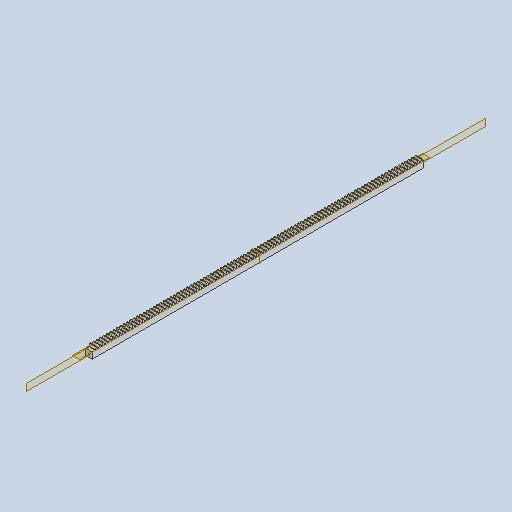
# Autodesk Inventor part: Zahnradbahn
Saved by Autodesk Inventor 2024 (Build 280153000, 153)
## iProperties
Created: 2022-05-05
Part Number: Zahnradbahn
Material: Generisch
Document SubType Name: Modeling
Designer: 123St
Density: 1 g/cm^3
Appearance: Vorgabe
Mass: 12.6552 g
Surface Area: 103.602 cm^2
Volume: 12.6552 cm^3
Zahnbreite: 1,700 mm
Teilung: 3,142 mm
Fussrundung: 0,380 mm
Modul: 1,000 mm
Kopfspiel: 0,100 mm
Zaehnezahl_1: 98,000 oE
Author: 123St
Autodesk Inventor part; units mm, degrees
(part 1 of 2)
ref_plane "YZ Plane" through (0, 0, 0) normal (1, 0, 0) x (0, 1, 0)
ref_plane "XZ Plane" through (0, 0, 0) normal (0, 1, 0) x (-1, 0, 0)
sketch "Skizze1" plane through (0, 0, 0) normal (1, 0, 0) x (0, 1, 0)
  line L0 (3.4, 153.938) -> (-3.4, 153.938)
  line L1 (-3.4, 153.938) -> (-3.4, -153.938)
  line L2 (-3.4, -153.938) -> (3.4, -153.938)
  line L3 (3.4, -153.938) -> (3.4, 153.938)
  line L4 (3.4, 153.938) -> (-3.4, -153.938) construction
  line L5 (-3.4, 153.938) -> (3.4, -153.938) construction
  point P0 (0, 0)
  dimension "d0" = 6.8
  dimension "d1" = 307.8761
  constraints: 12 end point, 2 midpoint, 2 parallel, 1 horizontal, 1 perpendicular
  measures "d0" distance of L0.start L0.end
  measures "d1" distance of L2.end L0.start
extrude "Extrusion1" add sketch "Skizze1" along normal blind 6
sketch "Skizze3" plane through (0, -3.4, -153.938) normal (0, -1, 0) x (1, 0, 0)
  line L0 (0, 307.8761) -> (6, 307.8761)
  line L1 (6, 307.8761) -> (6, 0)
  line L2 (6, 0) -> (0, 0)
  line L3 (0, 0) -> (0, 307.8761)
  line L4 (6, 307.8761) -> (6, 0) construction
  line L5 (0, 307.8761) -> (6, 307.8761) projected
  line L6 (0, 0) -> (0, 307.8761) construction
  line L7 (6, 0) -> (6, 307.8761) construction
  point P0 (0, 153.938)
  dimension "d21" = 307.8761
  dimension "d24" = 0
  constraints: 8 end point, 2 collinear, 2 parallel, 1 horizontal, 1 perpendicular
  measures "d21" distance of L0.end L1.end
  measures "d24" distance between parallel lines of L5 L0
extrude "Extrusion3" add sketch "Skizze3" along normal blind 2.5
sketch "Skizze5" plane through (6, 0, 0) normal (1, 0, 0) x (0, 0, -1)
  line L0 (-153.938, 3.4) -> (-153.938, -5.9) construction
  line L1 (-153.938, 0) -> (153.938, 0) construction
  line L2 (153.938, -5.9) -> (-153.938, -5.9) construction
  line L3 (-153.938, 0) -> (-153.686, 0)
  arc A0 (-153.686, 0) -> (-153.5075, 0.125) centre (-153.686, 0.19) ccw
  line L4 (-153.5075, 0.125) -> (-152.7887, 2.1)
  line L5 (-152.7887, 2.1) -> (-151.9458, 2.1)
  line L6 (-151.9458, 2.1) -> (-151.227, 0.125)
  arc A1 (-151.227, 0.125) -> (-151.0484, 0) centre (-151.0484, 0.19) ccw
  line L7 (-151.0484, 0) -> (-150.7964, 0)
  line L8 (-152.3672, 2.1) -> (-152.3672, 0) construction
  line L9 (-153.686, 0) -> (-151.0484, 0) construction
  line L10 (-153.1526, 1.1) -> (-151.5818, 1.1) construction
  line L11 (-147.9068, 0) -> (-147.6549, 0)
  arc A2 (-148.0854, 0.125) -> (-147.9068, 0) centre (-147.9068, 0.19) ccw
  line L12 (-150.011, 1.1) -> (-148.4403, 1.1) construction
  line L13 (-150.3659, 0.125) -> (-149.6471, 2.1)
  line L14 (-148.8042, 2.1) -> (-148.0854, 0.125)
  line L15 (-149.2257, 2.1) -> (-149.2257, 0) construction
  line L16 (-149.6471, 2.1) -> (-148.8042, 2.1)
  line L17 (-150.5445, 0) -> (-147.9068, 0) construction
  arc A3 (-150.5445, 0) -> (-150.3659, 0.125) centre (-150.5445, 0.19) ccw
  line L18 (-150.7964, 0) -> (-150.5445, 0)
  line L19 (-144.7653, 0) -> (-144.5133, 0)
  arc A4 (-144.9438, 0.125) -> (-144.7653, 0) centre (-144.7653, 0.19) ccw
  line L20 (-146.8695, 1.1) -> (-145.2987, 1.1) construction
  line L21 (-147.2243, 0.125) -> (-146.5055, 2.1)
  line L22 (-145.6626, 2.1) -> (-144.9438, 0.125)
  line L23 (-146.0841, 2.1) -> (-146.0841, 0) construction
  line L24 (-146.5055, 2.1) -> (-145.6626, 2.1)
  line L25 (-147.4029, 0) -> (-144.7653, 0) construction
  arc A5 (-147.4029, 0) -> (-147.2243, 0.125) centre (-147.4029, 0.19) ccw
  line L26 (-147.6549, 0) -> (-147.4029, 0)
  line L27 (-141.6237, 0) -> (-141.3717, 0)
  arc A6 (-141.8022, 0.125) -> (-141.6237, 0) centre (-141.6237, 0.19) ccw
  line L28 (-143.7279, 1.1) -> (-142.1571, 1.1) construction
  line L29 (-144.0827, 0.125) -> (-143.3639, 2.1)
  line L30 (-142.521, 2.1) -> (-141.8022, 0.125)
  line L31 (-142.9425, 2.1) -> (-142.9425, 0) construction
  line L32 (-143.3639, 2.1) -> (-142.521, 2.1)
  line L33 (-144.2613, 0) -> (-141.6237, 0) construction
  arc A7 (-144.2613, 0) -> (-144.0827, 0.125) centre (-144.2613, 0.19) ccw
  line L34 (-144.5133, 0) -> (-144.2613, 0)
  line L35 (-138.4821, 0) -> (-138.2301, 0)
  arc A8 (-138.6606, 0.125) -> (-138.4821, 0) centre (-138.4821, 0.19) ccw
  line L36 (-140.5863, 1.1) -> (-139.0155, 1.1) construction
  line L37 (-140.9411, 0.125) -> (-140.2223, 2.1)
  line L38 (-139.3794, 2.1) -> (-138.6606, 0.125)
  line L39 (-139.8009, 2.1) -> (-139.8009, 0) construction
  line L40 (-140.2223, 2.1) -> (-139.3794, 2.1)
  line L41 (-141.1197, 0) -> (-138.4821, 0) construction
  arc A9 (-141.1197, 0) -> (-140.9411, 0.125) centre (-141.1197, 0.19) ccw
  line L42 (-141.3717, 0) -> (-141.1197, 0)
  line L43 (-135.3405, 0) -> (-135.0885, 0)
  arc A10 (-135.519, 0.125) -> (-135.3405, 0) centre (-135.3405, 0.19) ccw
  line L44 (-137.4447, 1.1) -> (-135.8739, 1.1) construction
  line L45 (-137.7995, 0.125) -> (-137.0807, 2.1)
  line L46 (-136.2379, 2.1) -> (-135.519, 0.125)
  line L47 (-136.6593, 2.1) -> (-136.6593, 0) construction
  line L48 (-137.0807, 2.1) -> (-136.2379, 2.1)
  line L49 (-137.9781, 0) -> (-135.3405, 0) construction
  arc A11 (-137.9781, 0) -> (-137.7995, 0.125) centre (-137.9781, 0.19) ccw
  line L50 (-138.2301, 0) -> (-137.9781, 0)
  line L51 (-132.1989, 0) -> (-131.9469, 0)
  arc A12 (-132.3774, 0.125) -> (-132.1989, 0) centre (-132.1989, 0.19) ccw
  line L52 (-134.3031, 1.1) -> (-132.7323, 1.1) construction
  line L53 (-134.658, 0.125) -> (-133.9391, 2.1)
  line L54 (-133.0963, 2.1) -> (-132.3774, 0.125)
  line L55 (-133.5177, 2.1) -> (-133.5177, 0) construction
  line L56 (-133.9391, 2.1) -> (-133.0963, 2.1)
  line L57 (-134.8365, 0) -> (-132.1989, 0) construction
  arc A13 (-134.8365, 0) -> (-134.658, 0.125) centre (-134.8365, 0.19) ccw
  line L58 (-135.0885, 0) -> (-134.8365, 0)
  line L59 (-129.0573, 0) -> (-128.8053, 0)
  arc A14 (-129.2358, 0.125) -> (-129.0573, 0) centre (-129.0573, 0.19) ccw
  line L60 (-131.1615, 1.1) -> (-129.5907, 1.1) construction
  line L61 (-131.5164, 0.125) -> (-130.7975, 2.1)
  line L62 (-129.9547, 2.1) -> (-129.2358, 0.125)
  line L63 (-130.3761, 2.1) -> (-130.3761, 0) construction
  line L64 (-130.7975, 2.1) -> (-129.9547, 2.1)
  line L65 (-131.6949, 0) -> (-129.0573, 0) construction
  arc A15 (-131.6949, 0) -> (-131.5164, 0.125) centre (-131.6949, 0.19) ccw
  line L66 (-131.9469, 0) -> (-131.6949, 0)
  line L67 (-125.9157, 0) -> (-125.6637, 0)
  arc A16 (-126.0942, 0.125) -> (-125.9157, 0) centre (-125.9157, 0.19) ccw
  line L68 (-128.0199, 1.1) -> (-126.4491, 1.1) construction
  line L69 (-128.3748, 0.125) -> (-127.6559, 2.1)
  line L70 (-126.8131, 2.1) -> (-126.0942, 0.125)
  line L71 (-127.2345, 2.1) -> (-127.2345, 0) construction
  line L72 (-127.6559, 2.1) -> (-126.8131, 2.1)
  line L73 (-128.5533, 0) -> (-125.9157, 0) construction
  arc A17 (-128.5533, 0) -> (-128.3748, 0.125) centre (-128.5533, 0.19) ccw
  line L74 (-128.8053, 0) -> (-128.5533, 0)
  line L75 (-122.7741, 0) -> (-122.5221, 0)
  arc A18 (-122.9526, 0.125) -> (-122.7741, 0) centre (-122.7741, 0.19) ccw
  line L76 (-124.8783, 1.1) -> (-123.3075, 1.1) construction
  line L77 (-125.2332, 0.125) -> (-124.5143, 2.1)
  line L78 (-123.6715, 2.1) -> (-122.9526, 0.125)
  line L79 (-124.0929, 2.1) -> (-124.0929, 0) construction
  line L80 (-124.5143, 2.1) -> (-123.6715, 2.1)
  line L81 (-125.4117, 0) -> (-122.7741, 0) construction
  arc A19 (-125.4117, 0) -> (-125.2332, 0.125) centre (-125.4117, 0.19) ccw
  line L82 (-125.6637, 0) -> (-125.4117, 0)
  line L83 (-119.6325, 0) -> (-119.3805, 0)
  arc A20 (-119.8111, 0.125) -> (-119.6325, 0) centre (-119.6325, 0.19) ccw
  line L84 (-121.7367, 1.1) -> (-120.1659, 1.1) construction
  line L85 (-122.0916, 0.125) -> (-121.3727, 2.1)
  line L86 (-120.5299, 2.1) -> (-119.8111, 0.125)
  line L87 (-120.9513, 2.1) -> (-120.9513, 0) construction
  line L88 (-121.3727, 2.1) -> (-120.5299, 2.1)
  line L89 (-122.2701, 0) -> (-119.6325, 0) construction
  arc A21 (-122.2701, 0) -> (-122.0916, 0.125) centre (-122.2701, 0.19) ccw
  line L90 (-122.5221, 0) -> (-122.2701, 0)
  line L91 (-116.4909, 0) -> (-116.2389, 0)
  arc A22 (-116.6695, 0.125) -> (-116.4909, 0) centre (-116.4909, 0.19) ccw
  line L92 (-118.5951, 1.1) -> (-117.0243, 1.1) construction
  line L93 (-118.95, 0.125) -> (-118.2312, 2.1)
  line L94 (-117.3883, 2.1) -> (-116.6695, 0.125)
  line L95 (-117.8097, 2.1) -> (-117.8097, 0) construction
  line L96 (-118.2312, 2.1) -> (-117.3883, 2.1)
  line L97 (-119.1285, 0) -> (-116.4909, 0) construction
  arc A23 (-119.1285, 0) -> (-118.95, 0.125) centre (-119.1285, 0.19) ccw
  line L98 (-119.3805, 0) -> (-119.1285, 0)
  line L99 (-113.3493, 0) -> (-113.0973, 0)
  arc A24 (-113.5279, 0.125) -> (-113.3493, 0) centre (-113.3493, 0.19) ccw
  line L100 (-115.4535, 1.1) -> (-113.8827, 1.1) construction
  line L101 (-115.8084, 0.125) -> (-115.0896, 2.1)
  line L102 (-114.2467, 2.1) -> (-113.5279, 0.125)
  line L103 (-114.6681, 2.1) -> (-114.6681, 0) construction
  line L104 (-115.0896, 2.1) -> (-114.2467, 2.1)
  line L105 (-115.9869, 0) -> (-113.3493, 0) construction
  arc A25 (-115.9869, 0) -> (-115.8084, 0.125) centre (-115.9869, 0.19) ccw
  line L106 (-116.2389, 0) -> (-115.9869, 0)
  line L107 (-110.2077, 0) -> (-109.9557, 0)
  arc A26 (-110.3863, 0.125) -> (-110.2077, 0) centre (-110.2077, 0.19) ccw
  line L108 (-112.3119, 1.1) -> (-110.7411, 1.1) construction
  line L109 (-112.6668, 0.125) -> (-111.948, 2.1)
  line L110 (-111.1051, 2.1) -> (-110.3863, 0.125)
  line L111 (-111.5265, 2.1) -> (-111.5265, 0) construction
  line L112 (-111.948, 2.1) -> (-111.1051, 2.1)
  line L113 (-112.8453, 0) -> (-110.2077, 0) construction
  arc A27 (-112.8453, 0) -> (-112.6668, 0.125) centre (-112.8453, 0.19) ccw
  line L114 (-113.0973, 0) -> (-112.8453, 0)
  line L115 (-107.0661, 0) -> (-106.8142, 0)
  arc A28 (-107.2447, 0.125) -> (-107.0661, 0) centre (-107.0661, 0.19) ccw
  line L116 (-109.1703, 1.1) -> (-107.5995, 1.1) construction
  line L117 (-109.5252, 0.125) -> (-108.8064, 2.1)
  line L118 (-107.9635, 2.1) -> (-107.2447, 0.125)
  line L119 (-108.3849, 2.1) -> (-108.3849, 0) construction
  line L120 (-108.8064, 2.1) -> (-107.9635, 2.1)
  line L121 (-109.7038, 0) -> (-107.0661, 0) construction
  arc A29 (-109.7038, 0) -> (-109.5252, 0.125) centre (-109.7038, 0.19) ccw
  line L122 (-109.9557, 0) -> (-109.7038, 0)
  line L123 (-103.9245, 0) -> (-103.6726, 0)
  arc A30 (-104.1031, 0.125) -> (-103.9245, 0) centre (-103.9245, 0.19) ccw
  line L124 (-106.0288, 1.1) -> (-104.458, 1.1) construction
  line L125 (-106.3836, 0.125) -> (-105.6648, 2.1)
  line L126 (-104.8219, 2.1) -> (-104.1031, 0.125)
  line L127 (-105.2434, 2.1) -> (-105.2434, 0) construction
  line L128 (-105.6648, 2.1) -> (-104.8219, 2.1)
  line L129 (-106.5622, 0) -> (-103.9245, 0) construction
  arc A31 (-106.5622, 0) -> (-106.3836, 0.125) centre (-106.5622, 0.19) ccw
  line L130 (-106.8142, 0) -> (-106.5622, 0)
  line L131 (-100.783, 0) -> (-100.531, 0)
  arc A32 (-100.9615, 0.125) -> (-100.783, 0) centre (-100.783, 0.19) ccw
  line L132 (-102.8872, 1.1) -> (-101.3164, 1.1) construction
  line L133 (-103.242, 0.125) -> (-102.5232, 2.1)
  line L134 (-101.6803, 2.1) -> (-100.9615, 0.125)
  line L135 (-102.1018, 2.1) -> (-102.1018, 0) construction
  line L136 (-102.5232, 2.1) -> (-101.6803, 2.1)
  line L137 (-103.4206, 0) -> (-100.783, 0) construction
  arc A33 (-103.4206, 0) -> (-103.242, 0.125) centre (-103.4206, 0.19) ccw
  line L138 (-103.6726, 0) -> (-103.4206, 0)
  line L139 (-97.6414, 0) -> (-97.3894, 0)
  arc A34 (-97.8199, 0.125) -> (-97.6414, 0) centre (-97.6414, 0.19) ccw
  line L140 (-99.7456, 1.1) -> (-98.1748, 1.1) construction
  line L141 (-100.1004, 0.125) -> (-99.3816, 2.1)
  line L142 (-98.5387, 2.1) -> (-97.8199, 0.125)
  line L143 (-98.9602, 2.1) -> (-98.9602, 0) construction
  line L144 (-99.3816, 2.1) -> (-98.5387, 2.1)
  line L145 (-100.279, 0) -> (-97.6414, 0) construction
  arc A35 (-100.279, 0) -> (-100.1004, 0.125) centre (-100.279, 0.19) ccw
  line L146 (-100.531, 0) -> (-100.279, 0)
  line L147 (-94.4998, 0) -> (-94.2478, 0)
  arc A36 (-94.6783, 0.125) -> (-94.4998, 0) centre (-94.4998, 0.19) ccw
  line L148 (-96.604, 1.1) -> (-95.0332, 1.1) construction
  line L149 (-96.9588, 0.125) -> (-96.24, 2.1)
  line L150 (-95.3971, 2.1) -> (-94.6783, 0.125)
  line L151 (-95.8186, 2.1) -> (-95.8186, 0) construction
  line L152 (-96.24, 2.1) -> (-95.3971, 2.1)
  line L153 (-97.1374, 0) -> (-94.4998, 0) construction
  arc A37 (-97.1374, 0) -> (-96.9588, 0.125) centre (-97.1374, 0.19) ccw
  line L154 (-97.3894, 0) -> (-97.1374, 0)
  line L155 (-91.3582, 0) -> (-91.1062, 0)
  arc A38 (-91.5367, 0.125) -> (-91.3582, 0) centre (-91.3582, 0.19) ccw
  line L156 (-93.4624, 1.1) -> (-91.8916, 1.1) construction
  line L157 (-93.8172, 0.125) -> (-93.0984, 2.1)
  line L158 (-92.2556, 2.1) -> (-91.5367, 0.125)
  line L159 (-92.677, 2.1) -> (-92.677, 0) construction
  line L160 (-93.0984, 2.1) -> (-92.2556, 2.1)
  line L161 (-93.9958, 0) -> (-91.3582, 0) construction
  arc A39 (-93.9958, 0) -> (-93.8172, 0.125) centre (-93.9958, 0.19) ccw
  line L162 (-94.2478, 0) -> (-93.9958, 0)
  line L163 (-88.2166, 0) -> (-87.9646, 0)
  arc A40 (-88.3951, 0.125) -> (-88.2166, 0) centre (-88.2166, 0.19) ccw
  line L164 (-90.3208, 1.1) -> (-88.75, 1.1) construction
  line L165 (-90.6757, 0.125) -> (-89.9568, 2.1)
  line L166 (-89.114, 2.1) -> (-88.3951, 0.125)
  line L167 (-89.5354, 2.1) -> (-89.5354, 0) construction
  line L168 (-89.9568, 2.1) -> (-89.114, 2.1)
  line L169 (-90.8542, 0) -> (-88.2166, 0) construction
  arc A41 (-90.8542, 0) -> (-90.6757, 0.125) centre (-90.8542, 0.19) ccw
  line L170 (-91.1062, 0) -> (-90.8542, 0)
  line L171 (-85.075, 0) -> (-84.823, 0)
  arc A42 (-85.2535, 0.125) -> (-85.075, 0) centre (-85.075, 0.19) ccw
  line L172 (-87.1792, 1.1) -> (-85.6084, 1.1) construction
  line L173 (-87.5341, 0.125) -> (-86.8152, 2.1)
  line L174 (-85.9724, 2.1) -> (-85.2535, 0.125)
  line L175 (-86.3938, 2.1) -> (-86.3938, 0) construction
  line L176 (-86.8152, 2.1) -> (-85.9724, 2.1)
  line L177 (-87.7126, 0) -> (-85.075, 0) construction
  arc A43 (-87.7126, 0) -> (-87.5341, 0.125) centre (-87.7126, 0.19) ccw
  line L178 (-87.9646, 0) -> (-87.7126, 0)
  line L179 (-81.9334, 0) -> (-81.6814, 0)
  arc A44 (-82.1119, 0.125) -> (-81.9334, 0) centre (-81.9334, 0.19) ccw
  line L180 (-84.0376, 1.1) -> (-82.4668, 1.1) construction
  line L181 (-84.3925, 0.125) -> (-83.6736, 2.1)
  line L182 (-82.8308, 2.1) -> (-82.1119, 0.125)
  line L183 (-83.2522, 2.1) -> (-83.2522, 0) construction
  line L184 (-83.6736, 2.1) -> (-82.8308, 2.1)
  line L185 (-84.571, 0) -> (-81.9334, 0) construction
  arc A45 (-84.571, 0) -> (-84.3925, 0.125) centre (-84.571, 0.19) ccw
  line L186 (-84.823, 0) -> (-84.571, 0)
  line L187 (-78.7918, 0) -> (-78.5398, 0)
  arc A46 (-78.9703, 0.125) -> (-78.7918, 0) centre (-78.7918, 0.19) ccw
  line L188 (-80.896, 1.1) -> (-79.3252, 1.1) construction
  line L189 (-81.2509, 0.125) -> (-80.532, 2.1)
  line L190 (-79.6892, 2.1) -> (-78.9703, 0.125)
  line L191 (-80.1106, 2.1) -> (-80.1106, 0) construction
  line L192 (-80.532, 2.1) -> (-79.6892, 2.1)
  line L193 (-81.4294, 0) -> (-78.7918, 0) construction
  arc A47 (-81.4294, 0) -> (-81.2509, 0.125) centre (-81.4294, 0.19) ccw
  line L194 (-81.6814, 0) -> (-81.4294, 0)
  line L195 (-75.6502, 0) -> (-75.3982, 0)
  arc A48 (-75.8288, 0.125) -> (-75.6502, 0) centre (-75.6502, 0.19) ccw
  line L196 (-77.7544, 1.1) -> (-76.1836, 1.1) construction
  line L197 (-78.1093, 0.125) -> (-77.3904, 2.1)
  line L198 (-76.5476, 2.1) -> (-75.8288, 0.125)
  line L199 (-76.969, 2.1) -> (-76.969, 0) construction
  line L200 (-77.3904, 2.1) -> (-76.5476, 2.1)
  line L201 (-78.2878, 0) -> (-75.6502, 0) construction
  arc A49 (-78.2878, 0) -> (-78.1093, 0.125) centre (-78.2878, 0.19) ccw
  line L202 (-78.5398, 0) -> (-78.2878, 0)
  line L203 (-72.5086, 0) -> (-72.2566, 0)
  arc A50 (-72.6872, 0.125) -> (-72.5086, 0) centre (-72.5086, 0.19) ccw
  line L204 (-74.6128, 1.1) -> (-73.042, 1.1) construction
  line L205 (-74.9677, 0.125) -> (-74.2489, 2.1)
  line L206 (-73.406, 2.1) -> (-72.6872, 0.125)
  line L207 (-73.8274, 2.1) -> (-73.8274, 0) construction
  line L208 (-74.2489, 2.1) -> (-73.406, 2.1)
  line L209 (-75.1462, 0) -> (-72.5086, 0) construction
  arc A51 (-75.1462, 0) -> (-74.9677, 0.125) centre (-75.1462, 0.19) ccw
  line L210 (-75.3982, 0) -> (-75.1462, 0)
  line L211 (-69.367, 0) -> (-69.115, 0)
  arc A52 (-69.5456, 0.125) -> (-69.367, 0) centre (-69.367, 0.19) ccw
  line L212 (-71.4712, 1.1) -> (-69.9004, 1.1) construction
  line L213 (-71.8261, 0.125) -> (-71.1073, 2.1)
  line L214 (-70.2644, 2.1) -> (-69.5456, 0.125)
  line L215 (-70.6858, 2.1) -> (-70.6858, 0) construction
  line L216 (-71.1073, 2.1) -> (-70.2644, 2.1)
  line L217 (-72.0046, 0) -> (-69.367, 0) construction
  arc A53 (-72.0046, 0) -> (-71.8261, 0.125) centre (-72.0046, 0.19) ccw
  line L218 (-72.2566, 0) -> (-72.0046, 0)
  line L219 (-66.2254, 0) -> (-65.9734, 0)
  arc A54 (-66.404, 0.125) -> (-66.2254, 0) centre (-66.2254, 0.19) ccw
  line L220 (-68.3296, 1.1) -> (-66.7588, 1.1) construction
  line L221 (-68.6845, 0.125) -> (-67.9657, 2.1)
  line L222 (-67.1228, 2.1) -> (-66.404, 0.125)
  line L223 (-67.5442, 2.1) -> (-67.5442, 0) construction
  line L224 (-67.9657, 2.1) -> (-67.1228, 2.1)
  line L225 (-68.863, 0) -> (-66.2254, 0) construction
  arc A55 (-68.863, 0) -> (-68.6845, 0.125) centre (-68.863, 0.19) ccw
  line L226 (-69.115, 0) -> (-68.863, 0)
  line L227 (-63.0838, 0) -> (-62.8319, 0)
  arc A56 (-63.2624, 0.125) -> (-63.0838, 0) centre (-63.0838, 0.19) ccw
  line L228 (-65.188, 1.1) -> (-63.6173, 1.1) construction
  line L229 (-65.5429, 0.125) -> (-64.8241, 2.1)
  line L230 (-63.9812, 2.1) -> (-63.2624, 0.125)
  line L231 (-64.4026, 2.1) -> (-64.4026, 0) construction
  line L232 (-64.8241, 2.1) -> (-63.9812, 2.1)
  line L233 (-65.7215, 0) -> (-63.0838, 0) construction
  arc A57 (-65.7215, 0) -> (-65.5429, 0.125) centre (-65.7215, 0.19) ccw
  line L234 (-65.9734, 0) -> (-65.7215, 0)
  line L235 (-59.9423, 0) -> (-59.6903, 0)
  arc A58 (-60.1208, 0.125) -> (-59.9423, 0) centre (-59.9423, 0.19) ccw
  line L236 (-62.0465, 1.1) -> (-60.4757, 1.1) construction
  line L237 (-62.4013, 0.125) -> (-61.6825, 2.1)
  line L238 (-60.8396, 2.1) -> (-60.1208, 0.125)
  line L239 (-61.2611, 2.1) -> (-61.2611, 0) construction
  line L240 (-61.6825, 2.1) -> (-60.8396, 2.1)
  line L241 (-62.5799, 0) -> (-59.9423, 0) construction
  arc A59 (-62.5799, 0) -> (-62.4013, 0.125) centre (-62.5799, 0.19) ccw
  line L242 (-62.8319, 0) -> (-62.5799, 0)
  line L243 (-56.8007, 0) -> (-56.5487, 0)
  arc A60 (-56.9792, 0.125) -> (-56.8007, 0) centre (-56.8007, 0.19) ccw
  line L244 (-58.9049, 1.1) -> (-57.3341, 1.1) construction
  line L245 (-59.2597, 0.125) -> (-58.5409, 2.1)
  line L246 (-57.698, 2.1) -> (-56.9792, 0.125)
  line L247 (-58.1195, 2.1) -> (-58.1195, 0) construction
  line L248 (-58.5409, 2.1) -> (-57.698, 2.1)
  line L249 (-59.4383, 0) -> (-56.8007, 0) construction
  arc A61 (-59.4383, 0) -> (-59.2597, 0.125) centre (-59.4383, 0.19) ccw
  line L250 (-59.6903, 0) -> (-59.4383, 0)
  line L251 (-53.6591, 0) -> (-53.4071, 0)
  arc A62 (-53.8376, 0.125) -> (-53.6591, 0) centre (-53.6591, 0.19) ccw
  line L252 (-55.7633, 1.1) -> (-54.1925, 1.1) construction
  line L253 (-56.1181, 0.125) -> (-55.3993, 2.1)
  line L254 (-54.5564, 2.1) -> (-53.8376, 0.125)
  line L255 (-54.9779, 2.1) -> (-54.9779, 0) construction
  line L256 (-55.3993, 2.1) -> (-54.5564, 2.1)
  line L257 (-56.2967, 0) -> (-53.6591, 0) construction
  arc A63 (-56.2967, 0) -> (-56.1181, 0.125) centre (-56.2967, 0.19) ccw
  line L258 (-56.5487, 0) -> (-56.2967, 0)
  line L259 (-50.5175, 0) -> (-50.2655, 0)
  arc A64 (-50.696, 0.125) -> (-50.5175, 0) centre (-50.5175, 0.19) ccw
  line L260 (-52.6217, 1.1) -> (-51.0509, 1.1) construction
  line L261 (-52.9765, 0.125) -> (-52.2577, 2.1)
  line L262 (-51.4149, 2.1) -> (-50.696, 0.125)
  line L263 (-51.8363, 2.1) -> (-51.8363, 0) construction
  line L264 (-52.2577, 2.1) -> (-51.4149, 2.1)
  line L265 (-53.1551, 0) -> (-50.5175, 0) construction
  arc A65 (-53.1551, 0) -> (-52.9765, 0.125) centre (-53.1551, 0.19) ccw
  line L266 (-53.4071, 0) -> (-53.1551, 0)
  line L267 (-47.3759, 0) -> (-47.1239, 0)
  arc A66 (-47.5544, 0.125) -> (-47.3759, 0) centre (-47.3759, 0.19) ccw
  line L268 (-49.4801, 1.1) -> (-47.9093, 1.1) construction
  line L269 (-49.8349, 0.125) -> (-49.1161, 2.1)
  line L270 (-48.2733, 2.1) -> (-47.5544, 0.125)
  line L271 (-48.6947, 2.1) -> (-48.6947, 0) construction
  line L272 (-49.1161, 2.1) -> (-48.2733, 2.1)
  line L273 (-50.0135, 0) -> (-47.3759, 0) construction
  arc A67 (-50.0135, 0) -> (-49.8349, 0.125) centre (-50.0135, 0.19) ccw
  line L274 (-50.2655, 0) -> (-50.0135, 0)
  line L275 (-44.2343, 0) -> (-43.9823, 0)
  arc A68 (-44.4128, 0.125) -> (-44.2343, 0) centre (-44.2343, 0.19) ccw
  line L276 (-46.3385, 1.1) -> (-44.7677, 1.1) construction
  line L277 (-46.6934, 0.125) -> (-45.9745, 2.1)
  line L278 (-45.1317, 2.1) -> (-44.4128, 0.125)
  line L279 (-45.5531, 2.1) -> (-45.5531, 0) construction
  line L280 (-45.9745, 2.1) -> (-45.1317, 2.1)
  line L281 (-46.8719, 0) -> (-44.2343, 0) construction
  arc A69 (-46.8719, 0) -> (-46.6934, 0.125) centre (-46.8719, 0.19) ccw
  line L282 (-47.1239, 0) -> (-46.8719, 0)
  line L283 (-41.0927, 0) -> (-40.8407, 0)
  arc A70 (-41.2712, 0.125) -> (-41.0927, 0) centre (-41.0927, 0.19) ccw
  line L284 (-43.1969, 1.1) -> (-41.6261, 1.1) construction
  line L285 (-43.5518, 0.125) -> (-42.8329, 2.1)
  line L286 (-41.9901, 2.1) -> (-41.2712, 0.125)
  line L287 (-42.4115, 2.1) -> (-42.4115, 0) construction
  line L288 (-42.8329, 2.1) -> (-41.9901, 2.1)
  line L289 (-43.7303, 0) -> (-41.0927, 0) construction
  arc A71 (-43.7303, 0) -> (-43.5518, 0.125) centre (-43.7303, 0.19) ccw
  line L290 (-43.9823, 0) -> (-43.7303, 0)
  line L291 (-37.9511, 0) -> (-37.6991, 0)
  arc A72 (-38.1296, 0.125) -> (-37.9511, 0) centre (-37.9511, 0.19) ccw
  line L292 (-40.0553, 1.1) -> (-38.4845, 1.1) construction
  line L293 (-40.4102, 0.125) -> (-39.6913, 2.1)
  line L294 (-38.8485, 2.1) -> (-38.1296, 0.125)
  line L295 (-39.2699, 2.1) -> (-39.2699, 0) construction
  line L296 (-39.6913, 2.1) -> (-38.8485, 2.1)
  line L297 (-40.5887, 0) -> (-37.9511, 0) construction
  arc A73 (-40.5887, 0) -> (-40.4102, 0.125) centre (-40.5887, 0.19) ccw
  line L298 (-40.8407, 0) -> (-40.5887, 0)
  line L299 (-34.8095, 0) -> (-34.5575, 0)
  arc A74 (-34.9881, 0.125) -> (-34.8095, 0) centre (-34.8095, 0.19) ccw
  line L300 (-36.9137, 1.1) -> (-35.3429, 1.1) construction
  line L301 (-37.2686, 0.125) -> (-36.5497, 2.1)
  line L302 (-35.7069, 2.1) -> (-34.9881, 0.125)
  line L303 (-36.1283, 2.1) -> (-36.1283, 0) construction
  line L304 (-36.5497, 2.1) -> (-35.7069, 2.1)
  line L305 (-37.4471, 0) -> (-34.8095, 0) construction
  arc A75 (-37.4471, 0) -> (-37.2686, 0.125) centre (-37.4471, 0.19) ccw
  line L306 (-37.6991, 0) -> (-37.4471, 0)
  line L307 (-31.6679, 0) -> (-31.4159, 0)
  arc A76 (-31.8465, 0.125) -> (-31.6679, 0) centre (-31.6679, 0.19) ccw
  line L308 (-33.7721, 1.1) -> (-32.2013, 1.1) construction
  line L309 (-34.127, 0.125) -> (-33.4082, 2.1)
  line L310 (-32.5653, 2.1) -> (-31.8465, 0.125)
  line L311 (-32.9867, 2.1) -> (-32.9867, 0) construction
  line L312 (-33.4082, 2.1) -> (-32.5653, 2.1)
  line L313 (-34.3055, 0) -> (-31.6679, 0) construction
  arc A77 (-34.3055, 0) -> (-34.127, 0.125) centre (-34.3055, 0.19) ccw
  line L314 (-34.5575, 0) -> (-34.3055, 0)
  line L315 (-28.5263, 0) -> (-28.2743, 0)
  arc A78 (-28.7049, 0.125) -> (-28.5263, 0) centre (-28.5263, 0.19) ccw
  line L316 (-30.6305, 1.1) -> (-29.0597, 1.1) construction
  line L317 (-30.9854, 0.125) -> (-30.2666, 2.1)
  line L318 (-29.4237, 2.1) -> (-28.7049, 0.125)
  line L319 (-29.8451, 2.1) -> (-29.8451, 0) construction
  line L320 (-30.2666, 2.1) -> (-29.4237, 2.1)
  line L321 (-31.1639, 0) -> (-28.5263, 0) construction
  arc A79 (-31.1639, 0) -> (-30.9854, 0.125) centre (-31.1639, 0.19) ccw
  line L322 (-31.4159, 0) -> (-31.1639, 0)
  line L323 (-25.3847, 0) -> (-25.1327, 0)
  arc A80 (-25.5633, 0.125) -> (-25.3847, 0) centre (-25.3847, 0.19) ccw
  line L324 (-27.4889, 1.1) -> (-25.9181, 1.1) construction
  line L325 (-27.8438, 0.125) -> (-27.125, 2.1)
  line L326 (-26.2821, 2.1) -> (-25.5633, 0.125)
  line L327 (-26.7035, 2.1) -> (-26.7035, 0) construction
  line L328 (-27.125, 2.1) -> (-26.2821, 2.1)
  line L329 (-28.0223, 0) -> (-25.3847, 0) construction
  arc A81 (-28.0223, 0) -> (-27.8438, 0.125) centre (-28.0223, 0.19) ccw
  line L330 (-28.2743, 0) -> (-28.0223, 0)
  line L331 (-22.2431, 0) -> (-21.9911, 0)
  arc A82 (-22.4217, 0.125) -> (-22.2431, 0) centre (-22.2431, 0.19) ccw
  line L332 (-24.3473, 1.1) -> (-22.7765, 1.1) construction
  line L333 (-24.7022, 0.125) -> (-23.9834, 2.1)
  line L334 (-23.1405, 2.1) -> (-22.4217, 0.125)
  line L335 (-23.5619, 2.1) -> (-23.5619, 0) construction
  line L336 (-23.9834, 2.1) -> (-23.1405, 2.1)
  line L337 (-24.8807, 0) -> (-22.2431, 0) construction
  arc A83 (-24.8807, 0) -> (-24.7022, 0.125) centre (-24.8807, 0.19) ccw
  line L338 (-25.1327, 0) -> (-24.8807, 0)
  line L339 (-19.1015, 0) -> (-18.8496, 0)
  arc A84 (-19.2801, 0.125) -> (-19.1015, 0) centre (-19.1015, 0.19) ccw
  line L340 (-21.2058, 1.1) -> (-19.635, 1.1) construction
  line L341 (-21.5606, 0.125) -> (-20.8418, 2.1)
  line L342 (-19.9989, 2.1) -> (-19.2801, 0.125)
  line L343 (-20.4204, 2.1) -> (-20.4204, 0) construction
  line L344 (-20.8418, 2.1) -> (-19.9989, 2.1)
  line L345 (-21.7392, 0) -> (-19.1015, 0) construction
  arc A85 (-21.7392, 0) -> (-21.5606, 0.125) centre (-21.7392, 0.19) ccw
  line L346 (-21.9911, 0) -> (-21.7392, 0)
  line L347 (-15.96, 0) -> (-15.708, 0)
  arc A86 (-16.1385, 0.125) -> (-15.96, 0) centre (-15.96, 0.19) ccw
  line L348 (-18.0642, 1.1) -> (-16.4934, 1.1) construction
  line L349 (-18.419, 0.125) -> (-17.7002, 2.1)
  line L350 (-16.8573, 2.1) -> (-16.1385, 0.125)
  line L351 (-17.2788, 2.1) -> (-17.2788, 0) construction
  line L352 (-17.7002, 2.1) -> (-16.8573, 2.1)
  line L353 (-18.5976, 0) -> (-15.96, 0) construction
  arc A87 (-18.5976, 0) -> (-18.419, 0.125) centre (-18.5976, 0.19) ccw
  line L354 (-18.8496, 0) -> (-18.5976, 0)
  line L355 (-12.8184, 0) -> (-12.5664, 0)
  arc A88 (-12.9969, 0.125) -> (-12.8184, 0) centre (-12.8184, 0.19) ccw
  line L356 (-14.9226, 1.1) -> (-13.3518, 1.1) construction
  line L357 (-15.2774, 0.125) -> (-14.5586, 2.1)
  line L358 (-13.7157, 2.1) -> (-12.9969, 0.125)
  line L359 (-14.1372, 2.1) -> (-14.1372, 0) construction
  line L360 (-14.5586, 2.1) -> (-13.7157, 2.1)
  line L361 (-15.456, 0) -> (-12.8184, 0) construction
  arc A89 (-15.456, 0) -> (-15.2774, 0.125) centre (-15.456, 0.19) ccw
  line L362 (-15.708, 0) -> (-15.456, 0)
  line L363 (-9.6768, 0) -> (-9.4248, 0)
  arc A90 (-9.8553, 0.125) -> (-9.6768, 0) centre (-9.6768, 0.19) ccw
  line L364 (-11.781, 1.1) -> (-10.2102, 1.1) construction
  line L365 (-12.1358, 0.125) -> (-11.417, 2.1)
  line L366 (-10.5741, 2.1) -> (-9.8553, 0.125)
  line L367 (-10.9956, 2.1) -> (-10.9956, 0) construction
  line L368 (-11.417, 2.1) -> (-10.5741, 2.1)
  line L369 (-12.3144, 0) -> (-9.6768, 0) construction
  arc A91 (-12.3144, 0) -> (-12.1358, 0.125) centre (-12.3144, 0.19) ccw
  line L370 (-12.5664, 0) -> (-12.3144, 0)
  line L371 (-6.5352, 0) -> (-6.2832, 0)
  arc A92 (-6.7137, 0.125) -> (-6.5352, 0) centre (-6.5352, 0.19) ccw
  line L372 (-8.6394, 1.1) -> (-7.0686, 1.1) construction
  line L373 (-8.9942, 0.125) -> (-8.2754, 2.1)
  line L374 (-7.4326, 2.1) -> (-6.7137, 0.125)
  line L375 (-7.854, 2.1) -> (-7.854, 0) construction
  line L376 (-8.2754, 2.1) -> (-7.4326, 2.1)
  line L377 (-9.1728, 0) -> (-6.5352, 0) construction
  arc A93 (-9.1728, 0) -> (-8.9942, 0.125) centre (-9.1728, 0.19) ccw
  line L378 (-9.4248, 0) -> (-9.1728, 0)
  line L379 (-3.3936, 0) -> (-3.1416, 0)
  arc A94 (-3.5721, 0.125) -> (-3.3936, 0) centre (-3.3936, 0.19) ccw
  line L380 (-5.4978, 1.1) -> (-3.927, 1.1) construction
  line L381 (-5.8527, 0.125) -> (-5.1338, 2.1)
  line L382 (-4.291, 2.1) -> (-3.5721, 0.125)
  line L383 (-4.7124, 2.1) -> (-4.7124, 0) construction
  line L384 (-5.1338, 2.1) -> (-4.291, 2.1)
  line L385 (-6.0312, 0) -> (-3.3936, 0) construction
  arc A95 (-6.0312, 0) -> (-5.8527, 0.125) centre (-6.0312, 0.19) ccw
  line L386 (-6.2832, 0) -> (-6.0312, 0)
  line L387 (-0.252, 0) -> (0, 0)
  arc A96 (-0.4305, 0.125) -> (-0.252, 0) centre (-0.252, 0.19) ccw
  line L388 (-2.3562, 1.1) -> (-0.7854, 1.1) construction
  line L389 (-2.7111, 0.125) -> (-1.9922, 2.1)
  line L390 (-1.1494, 2.1) -> (-0.4305, 0.125)
  line L391 (-1.5708, 2.1) -> (-1.5708, 0) construction
  line L392 (-1.9922, 2.1) -> (-1.1494, 2.1)
  line L393 (-2.8896, 0) -> (-0.252, 0) construction
  arc A97 (-2.8896, 0) -> (-2.7111, 0.125) centre (-2.8896, 0.19) ccw
  line L394 (-3.1416, 0) -> (-2.8896, 0)
  line L395 (2.8896, 0) -> (3.1416, 0)
  arc A98 (2.7111, 0.125) -> (2.8896, 0) centre (2.8896, 0.19) ccw
  line L396 (0.7854, 1.1) -> (2.3562, 1.1) construction
  line L397 (0.4305, 0.125) -> (1.1494, 2.1)
  line L398 (1.9922, 2.1) -> (2.7111, 0.125)
  line L399 (1.5708, 2.1) -> (1.5708, 0) construction
  line L400 (1.1494, 2.1) -> (1.9922, 2.1)
  line L401 (0.252, 0) -> (2.8896, 0) construction
  arc A99 (0.252, 0) -> (0.4305, 0.125) centre (0.252, 0.19) ccw
  line L402 (0, 0) -> (0.252, 0)
  line L403 (6.0312, 0) -> (6.2832, 0)
  arc A100 (5.8527, 0.125) -> (6.0312, 0) centre (6.0312, 0.19) ccw
  line L404 (3.927, 1.1) -> (5.4978, 1.1) construction
  line L405 (3.5721, 0.125) -> (4.291, 2.1)
  line L406 (5.1338, 2.1) -> (5.8527, 0.125)
  line L407 (4.7124, 2.1) -> (4.7124, 0) construction
  line L408 (4.291, 2.1) -> (5.1338, 2.1)
  line L409 (3.3936, 0) -> (6.0312, 0) construction
  arc A101 (3.3936, 0) -> (3.5721, 0.125) centre (3.3936, 0.19) ccw
  line L410 (3.1416, 0) -> (3.3936, 0)
  line L411 (9.1728, 0) -> (9.4248, 0)
  arc A102 (8.9942, 0.125) -> (9.1728, 0) centre (9.1728, 0.19) ccw
  line L412 (7.0686, 1.1) -> (8.6394, 1.1) construction
  line L413 (6.7137, 0.125) -> (7.4326, 2.1)
  line L414 (8.2754, 2.1) -> (8.9942, 0.125)
  line L415 (7.854, 2.1) -> (7.854, 0) construction
  line L416 (7.4326, 2.1) -> (8.2754, 2.1)
  line L417 (6.5352, 0) -> (9.1728, 0) construction
  arc A103 (6.5352, 0) -> (6.7137, 0.125) centre (6.5352, 0.19) ccw
  line L418 (6.2832, 0) -> (6.5352, 0)
  line L419 (12.3144, 0) -> (12.5664, 0)
  arc A104 (12.1358, 0.125) -> (12.3144, 0) centre (12.3144, 0.19) ccw
  line L420 (10.2102, 1.1) -> (11.781, 1.1) construction
  line L421 (9.8553, 0.125) -> (10.5741, 2.1)
  line L422 (11.417, 2.1) -> (12.1358, 0.125)
  line L423 (10.9956, 2.1) -> (10.9956, 0) construction
  line L424 (10.5741, 2.1) -> (11.417, 2.1)
  line L425 (9.6768, 0) -> (12.3144, 0) construction
  arc A105 (9.6768, 0) -> (9.8553, 0.125) centre (9.6768, 0.19) ccw
  line L426 (9.4248, 0) -> (9.6768, 0)
  line L427 (15.456, 0) -> (15.708, 0)
  arc A106 (15.2774, 0.125) -> (15.456, 0) centre (15.456, 0.19) ccw
  line L428 (13.3518, 1.1) -> (14.9226, 1.1) construction
  line L429 (12.9969, 0.125) -> (13.7157, 2.1)
  line L430 (14.5586, 2.1) -> (15.2774, 0.125)
  line L431 (14.1372, 2.1) -> (14.1372, 0) construction
  line L432 (13.7157, 2.1) -> (14.5586, 2.1)
  line L433 (12.8184, 0) -> (15.456, 0) construction
  arc A107 (12.8184, 0) -> (12.9969, 0.125) centre (12.8184, 0.19) ccw
  line L434 (12.5664, 0) -> (12.8184, 0)
  line L435 (18.5976, 0) -> (18.8496, 0)
  arc A108 (18.419, 0.125) -> (18.5976, 0) centre (18.5976, 0.19) ccw
  line L436 (16.4934, 1.1) -> (18.0642, 1.1) construction
  line L437 (16.1385, 0.125) -> (16.8573, 2.1)
  line L438 (17.7002, 2.1) -> (18.419, 0.125)
  line L439 (17.2788, 2.1) -> (17.2788, 0) construction
  line L440 (16.8573, 2.1) -> (17.7002, 2.1)
  line L441 (15.96, 0) -> (18.5976, 0) construction
  arc A109 (15.96, 0) -> (16.1385, 0.125) centre (15.96, 0.19) ccw
  line L442 (15.708, 0) -> (15.96, 0)
  line L443 (21.7392, 0) -> (21.9911, 0)
  arc A110 (21.5606, 0.125) -> (21.7392, 0) centre (21.7392, 0.19) ccw
  line L444 (19.635, 1.1) -> (21.2058, 1.1) construction
  line L445 (19.2801, 0.125) -> (19.9989, 2.1)
  line L446 (20.8418, 2.1) -> (21.5606, 0.125)
  line L447 (20.4204, 2.1) -> (20.4204, 0) construction
  line L448 (19.9989, 2.1) -> (20.8418, 2.1)
  line L449 (19.1015, 0) -> (21.7392, 0) construction
  arc A111 (19.1015, 0) -> (19.2801, 0.125) centre (19.1015, 0.19) ccw
  line L450 (18.8496, 0) -> (19.1015, 0)
  line L451 (24.8807, 0) -> (25.1327, 0)
  arc A112 (24.7022, 0.125) -> (24.8807, 0) centre (24.8807, 0.19) ccw
  line L452 (22.7765, 1.1) -> (24.3473, 1.1) construction
  line L453 (22.4217, 0.125) -> (23.1405, 2.1)
  line L454 (23.9834, 2.1) -> (24.7022, 0.125)
  line L455 (23.5619, 2.1) -> (23.5619, 0) construction
  line L456 (23.1405, 2.1) -> (23.9834, 2.1)
  line L457 (22.2431, 0) -> (24.8807, 0) construction
  arc A113 (22.2431, 0) -> (22.4217, 0.125) centre (22.2431, 0.19) ccw
  line L458 (21.9911, 0) -> (22.2431, 0)
  line L459 (28.0223, 0) -> (28.2743, 0)
  arc A114 (27.8438, 0.125) -> (28.0223, 0) centre (28.0223, 0.19) ccw
  line L460 (25.9181, 1.1) -> (27.4889, 1.1) construction
  line L461 (25.5633, 0.125) -> (26.2821, 2.1)
  line L462 (27.125, 2.1) -> (27.8438, 0.125)
  line L463 (26.7035, 2.1) -> (26.7035, 0) construction
  line L464 (26.2821, 2.1) -> (27.125, 2.1)
  line L465 (25.3847, 0) -> (28.0223, 0) construction
  arc A115 (25.3847, 0) -> (25.5633, 0.125) centre (25.3847, 0.19) ccw
  line L466 (25.1327, 0) -> (25.3847, 0)
  line L467 (31.1639, 0) -> (31.4159, 0)
  arc A116 (30.9854, 0.125) -> (31.1639, 0) centre (31.1639, 0.19) ccw
  line L468 (29.0597, 1.1) -> (30.6305, 1.1) construction
  line L469 (28.7049, 0.125) -> (29.4237, 2.1)
  line L470 (30.2666, 2.1) -> (30.9854, 0.125)
  line L471 (29.8451, 2.1) -> (29.8451, 0) construction
  line L472 (29.4237, 2.1) -> (30.2666, 2.1)
  line L473 (28.5263, 0) -> (31.1639, 0) construction
  arc A117 (28.5263, 0) -> (28.7049, 0.125) centre (28.5263, 0.19) ccw
  line L474 (28.2743, 0) -> (28.5263, 0)
  line L475 (34.3055, 0) -> (34.5575, 0)
  arc A118 (34.127, 0.125) -> (34.3055, 0) centre (34.3055, 0.19) ccw
  line L476 (32.2013, 1.1) -> (33.7721, 1.1) construction
  line L477 (31.8465, 0.125) -> (32.5653, 2.1)
  line L478 (33.4082, 2.1) -> (34.127, 0.125)
  line L479 (32.9867, 2.1) -> (32.9867, 0) construction
  line L480 (32.5653, 2.1) -> (33.4082, 2.1)
  line L481 (31.6679, 0) -> (34.3055, 0) construction
  arc A119 (31.6679, 0) -> (31.8465, 0.125) centre (31.6679, 0.19) ccw
  line L482 (31.4159, 0) -> (31.6679, 0)
  line L483 (37.4471, 0) -> (37.6991, 0)
  arc A120 (37.2686, 0.125) -> (37.4471, 0) centre (37.4471, 0.19) ccw
  line L484 (35.3429, 1.1) -> (36.9137, 1.1) construction
  line L485 (34.9881, 0.125) -> (35.7069, 2.1)
  line L486 (36.5497, 2.1) -> (37.2686, 0.125)
  line L487 (36.1283, 2.1) -> (36.1283, 0) construction
  line L488 (35.7069, 2.1) -> (36.5497, 2.1)
  line L489 (34.8095, 0) -> (37.4471, 0) construction
  arc A121 (34.8095, 0) -> (34.9881, 0.125) centre (34.8095, 0.19) ccw
  line L490 (34.5575, 0) -> (34.8095, 0)
  line L491 (40.5887, 0) -> (40.8407, 0)
  arc A122 (40.4102, 0.125) -> (40.5887, 0) centre (40.5887, 0.19) ccw
  line L492 (38.4845, 1.1) -> (40.0553, 1.1) construction
  line L493 (38.1296, 0.125) -> (38.8485, 2.1)
  line L494 (39.6913, 2.1) -> (40.4102, 0.125)
  line L495 (39.2699, 2.1) -> (39.2699, 0) construction
  line L496 (38.8485, 2.1) -> (39.6913, 2.1)
  line L497 (37.9511, 0) -> (40.5887, 0) construction
  arc A123 (37.9511, 0) -> (38.1296, 0.125) centre (37.9511, 0.19) ccw
  line L498 (37.6991, 0) -> (37.9511, 0)
  line L499 (43.7303, 0) -> (43.9823, 0)
  arc A124 (43.5518, 0.125) -> (43.7303, 0) centre (43.7303, 0.19) ccw
  line L500 (41.6261, 1.1) -> (43.1969, 1.1) construction
  line L501 (41.2712, 0.125) -> (41.9901, 2.1)
  line L502 (42.8329, 2.1) -> (43.5518, 0.125)
  line L503 (42.4115, 2.1) -> (42.4115, 0) construction
  line L504 (41.9901, 2.1) -> (42.8329, 2.1)
  line L505 (41.0927, 0) -> (43.7303, 0) construction
  arc A125 (41.0927, 0) -> (41.2712, 0.125) centre (41.0927, 0.19) ccw
  line L506 (40.8407, 0) -> (41.0927, 0)
  line L507 (46.8719, 0) -> (47.1239, 0)
  arc A126 (46.6934, 0.125) -> (46.8719, 0) centre (46.8719, 0.19) ccw
  line L508 (44.7677, 1.1) -> (46.3385, 1.1) construction
  line L509 (44.4128, 0.125) -> (45.1317, 2.1)
  line L510 (45.9745, 2.1) -> (46.6934, 0.125)
  line L511 (45.5531, 2.1) -> (45.5531, 0) construction
  line L512 (45.1317, 2.1) -> (45.9745, 2.1)
  line L513 (44.2343, 0) -> (46.8719, 0) construction
  arc A127 (44.2343, 0) -> (44.4128, 0.125) centre (44.2343, 0.19) ccw
  line L514 (43.9823, 0) -> (44.2343, 0)
  line L515 (50.0135, 0) -> (50.2655, 0)
  arc A128 (49.8349, 0.125) -> (50.0135, 0) centre (50.0135, 0.19) ccw
  line L516 (47.9093, 1.1) -> (49.4801, 1.1) construction
  line L517 (47.5544, 0.125) -> (48.2733, 2.1)
  line L518 (49.1161, 2.1) -> (49.8349, 0.125)
  line L519 (48.6947, 2.1) -> (48.6947, 0) construction
  line L520 (48.2733, 2.1) -> (49.1161, 2.1)
  line L521 (47.3759, 0) -> (50.0135, 0) construction
  arc A129 (47.3759, 0) -> (47.5544, 0.125) centre (47.3759, 0.19) ccw
  line L522 (47.1239, 0) -> (47.3759, 0)
  line L523 (53.1551, 0) -> (53.4071, 0)
  arc A130 (52.9765, 0.125) -> (53.1551, 0) centre (53.1551, 0.19) ccw
  line L524 (51.0509, 1.1) -> (52.6217, 1.1) construction
  line L525 (50.696, 0.125) -> (51.4149, 2.1)
  line L526 (52.2577, 2.1) -> (52.9765, 0.125)
  line L527 (51.8363, 2.1) -> (51.8363, 0) construction
  line L528 (51.4149, 2.1) -> (52.2577, 2.1)
  line L529 (50.5175, 0) -> (53.1551, 0) construction
  arc A131 (50.5175, 0) -> (50.696, 0.125) centre (50.5175, 0.19) ccw
  line L530 (50.2655, 0) -> (50.5175, 0)
  line L531 (56.2967, 0) -> (56.5487, 0)
  arc A132 (56.1181, 0.125) -> (56.2967, 0) centre (56.2967, 0.19) ccw
  line L532 (54.1925, 1.1) -> (55.7633, 1.1) construction
  line L533 (53.8376, 0.125) -> (54.5564, 2.1)
  line L534 (55.3993, 2.1) -> (56.1181, 0.125)
  line L535 (54.9779, 2.1) -> (54.9779, 0) construction
  line L536 (54.5564, 2.1) -> (55.3993, 2.1)
  line L537 (53.6591, 0) -> (56.2967, 0) construction
  arc A133 (53.6591, 0) -> (53.8376, 0.125) centre (53.6591, 0.19) ccw
  line L538 (53.4071, 0) -> (53.6591, 0)
  line L539 (59.4383, 0) -> (59.6903, 0)
  arc A134 (59.2597, 0.125) -> (59.4383, 0) centre (59.4383, 0.19) ccw
  line L540 (57.3341, 1.1) -> (58.9049, 1.1) construction
  line L541 (56.9792, 0.125) -> (57.698, 2.1)
  line L542 (58.5409, 2.1) -> (59.2597, 0.125)
  line L543 (58.1195, 2.1) -> (58.1195, 0) construction
  line L544 (57.698, 2.1) -> (58.5409, 2.1)
  line L545 (56.8007, 0) -> (59.4383, 0) construction
  arc A135 (56.8007, 0) -> (56.9792, 0.125) centre (56.8007, 0.19) ccw
  line L546 (56.5487, 0) -> (56.8007, 0)
  line L547 (62.5799, 0) -> (62.8319, 0)
  arc A136 (62.4013, 0.125) -> (62.5799, 0) centre (62.5799, 0.19) ccw
  line L548 (60.4757, 1.1) -> (62.0465, 1.1) construction
  line L549 (60.1208, 0.125) -> (60.8396, 2.1)
  line L550 (61.6825, 2.1) -> (62.4013, 0.125)
  line L551 (61.2611, 2.1) -> (61.2611, 0) construction
  line L552 (60.8396, 2.1) -> (61.6825, 2.1)
  line L553 (59.9423, 0) -> (62.5799, 0) construction
  arc A137 (59.9423, 0) -> (60.1208, 0.125) centre (59.9423, 0.19) ccw
  line L554 (59.6903, 0) -> (59.9423, 0)
  line L555 (65.7215, 0) -> (65.9734, 0)
  arc A138 (65.5429, 0.125) -> (65.7215, 0) centre (65.7215, 0.19) ccw
  line L556 (63.6173, 1.1) -> (65.188, 1.1) construction
  line L557 (63.2624, 0.125) -> (63.9812, 2.1)
  line L558 (64.8241, 2.1) -> (65.5429, 0.125)
  line L559 (64.4026, 2.1) -> (64.4026, 0) construction
  line L560 (63.9812, 2.1) -> (64.8241, 2.1)
  line L561 (63.0838, 0) -> (65.7215, 0) construction
  arc A139 (63.0838, 0) -> (63.2624, 0.125) centre (63.0838, 0.19) ccw
  line L562 (62.8319, 0) -> (63.0838, 0)
  line L563 (68.863, 0) -> (69.115, 0)
  arc A140 (68.6845, 0.125) -> (68.863, 0) centre (68.863, 0.19) ccw
  line L564 (66.7588, 1.1) -> (68.3296, 1.1) construction
  line L565 (66.404, 0.125) -> (67.1228, 2.1)
  line L566 (67.9657, 2.1) -> (68.6845, 0.125)
  line L567 (67.5442, 2.1) -> (67.5442, 0) construction
  line L568 (67.1228, 2.1) -> (67.9657, 2.1)
  line L569 (66.2254, 0) -> (68.863, 0) construction
  arc A141 (66.2254, 0) -> (66.404, 0.125) centre (66.2254, 0.19) ccw
  line L570 (65.9734, 0) -> (66.2254, 0)
  line L571 (72.0046, 0) -> (72.2566, 0)
  arc A142 (71.8261, 0.125) -> (72.0046, 0) centre (72.0046, 0.19) ccw
  line L572 (69.9004, 1.1) -> (71.4712, 1.1) construction
  line L573 (69.5456, 0.125) -> (70.2644, 2.1)
  line L574 (71.1073, 2.1) -> (71.8261, 0.125)
  line L575 (70.6858, 2.1) -> (70.6858, 0) construction
  line L576 (70.2644, 2.1) -> (71.1073, 2.1)
  line L577 (69.367, 0) -> (72.0046, 0) construction
  arc A143 (69.367, 0) -> (69.5456, 0.125) centre (69.367, 0.19) ccw
  line L578 (69.115, 0) -> (69.367, 0)
  line L579 (75.1462, 0) -> (75.3982, 0)
  arc A144 (74.9677, 0.125) -> (75.1462, 0) centre (75.1462, 0.19) ccw
  line L580 (73.042, 1.1) -> (74.6128, 1.1) construction
  line L581 (72.6872, 0.125) -> (73.406, 2.1)
  line L582 (74.2489, 2.1) -> (74.9677, 0.125)
  line L583 (73.8274, 2.1) -> (73.8274, 0) construction
  line L584 (73.406, 2.1) -> (74.2489, 2.1)
  line L585 (72.5086, 0) -> (75.1462, 0) construction
  arc A145 (72.5086, 0) -> (72.6872, 0.125) centre (72.5086, 0.19) ccw
  line L586 (72.2566, 0) -> (72.5086, 0)
  line L587 (78.2878, 0) -> (78.5398, 0)
  arc A146 (78.1093, 0.125) -> (78.2878, 0) centre (78.2878, 0.19) ccw
  line L588 (76.1836, 1.1) -> (77.7544, 1.1) construction
  line L589 (75.8288, 0.125) -> (76.5476, 2.1)
  line L590 (77.3904, 2.1) -> (78.1093, 0.125)
  line L591 (76.969, 2.1) -> (76.969, 0) construction
  line L592 (76.5476, 2.1) -> (77.3904, 2.1)
  line L593 (75.6502, 0) -> (78.2878, 0) construction
  arc A147 (75.6502, 0) -> (75.8288, 0.125) centre (75.6502, 0.19) ccw
  line L594 (75.3982, 0) -> (75.6502, 0)
  line L595 (81.4294, 0) -> (81.6814, 0)
  arc A148 (81.2509, 0.125) -> (81.4294, 0) centre (81.4294, 0.19) ccw
  line L596 (79.3252, 1.1) -> (80.896, 1.1) construction
  line L597 (78.9703, 0.125) -> (79.6892, 2.1)
  line L598 (80.532, 2.1) -> (81.2509, 0.125)
  line L599 (80.1106, 2.1) -> (80.1106, 0) construction
  line L600 (79.6892, 2.1) -> (80.532, 2.1)
  line L601 (78.7918, 0) -> (81.4294, 0) construction
  arc A149 (78.7918, 0) -> (78.9703, 0.125) centre (78.7918, 0.19) ccw
  line L602 (78.5398, 0) -> (78.7918, 0)
  line L603 (84.571, 0) -> (84.823, 0)
  arc A150 (84.3925, 0.125) -> (84.571, 0) centre (84.571, 0.19) ccw
  line L604 (82.4668, 1.1) -> (84.0376, 1.1) construction
  line L605 (82.1119, 0.125) -> (82.8308, 2.1)
  line L606 (83.6736, 2.1) -> (84.3925, 0.125)
  line L607 (83.2522, 2.1) -> (83.2522, 0) construction
  line L608 (82.8308, 2.1) -> (83.6736, 2.1)
  line L609 (81.9334, 0) -> (84.571, 0) construction
  arc A151 (81.9334, 0) -> (82.1119, 0.125) centre (81.9334, 0.19) ccw
  line L610 (81.6814, 0) -> (81.9334, 0)
  line L611 (87.7126, 0) -> (87.9646, 0)
  arc A152 (87.5341, 0.125) -> (87.7126, 0) centre (87.7126, 0.19) ccw
  line L612 (85.6084, 1.1) -> (87.1792, 1.1) construction
  line L613 (85.2535, 0.125) -> (85.9724, 2.1)
  line L614 (86.8152, 2.1) -> (87.5341, 0.125)
  line L615 (86.3938, 2.1) -> (86.3938, 0) construction
  line L616 (85.9724, 2.1) -> (86.8152, 2.1)
  line L617 (85.075, 0) -> (87.7126, 0) construction
  arc A153 (85.075, 0) -> (85.2535, 0.125) centre (85.075, 0.19) ccw
  line L618 (84.823, 0) -> (85.075, 0)
  line L619 (90.8542, 0) -> (91.1062, 0)
  arc A154 (90.6757, 0.125) -> (90.8542, 0) centre (90.8542, 0.19) ccw
  line L620 (88.75, 1.1) -> (90.3208, 1.1) construction
  line L621 (88.3951, 0.125) -> (89.114, 2.1)
  line L622 (89.9568, 2.1) -> (90.6757, 0.125)
  line L623 (89.5354, 2.1) -> (89.5354, 0) construction
  line L624 (89.114, 2.1) -> (89.9568, 2.1)
  line L625 (88.2166, 0) -> (90.8542, 0) construction
  arc A155 (88.2166, 0) -> (88.3951, 0.125) centre (88.2166, 0.19) ccw
  line L626 (87.9646, 0) -> (88.2166, 0)
  line L627 (93.9958, 0) -> (94.2478, 0)
  arc A156 (93.8172, 0.125) -> (93.9958, 0) centre (93.9958, 0.19) ccw
  line L628 (91.8916, 1.1) -> (93.4624, 1.1) construction
  line L629 (91.5367, 0.125) -> (92.2556, 2.1)
  line L630 (93.0984, 2.1) -> (93.8172, 0.125)
  line L631 (92.677, 2.1) -> (92.677, 0) construction
  line L632 (92.2556, 2.1) -> (93.0984, 2.1)
  line L633 (91.3582, 0) -> (93.9958, 0) construction
  arc A157 (91.3582, 0) -> (91.5367, 0.125) centre (91.3582, 0.19) ccw
  line L634 (91.1062, 0) -> (91.3582, 0)
  line L635 (97.1374, 0) -> (97.3894, 0)
  arc A158 (96.9588, 0.125) -> (97.1374, 0) centre (97.1374, 0.19) ccw
  line L636 (95.0332, 1.1) -> (96.604, 1.1) construction
  line L637 (94.6783, 0.125) -> (95.3971, 2.1)
  line L638 (96.24, 2.1) -> (96.9588, 0.125)
  line L639 (95.8186, 2.1) -> (95.8186, 0) construction
  line L640 (95.3971, 2.1) -> (96.24, 2.1)
  line L641 (94.4998, 0) -> (97.1374, 0) construction
  arc A159 (94.4998, 0) -> (94.6783, 0.125) centre (94.4998, 0.19) ccw
  line L642 (94.2478, 0) -> (94.4998, 0)
  line L643 (100.279, 0) -> (100.531, 0)
  arc A160 (100.1004, 0.125) -> (100.279, 0) centre (100.279, 0.19) ccw
  line L644 (98.1748, 1.1) -> (99.7456, 1.1) construction
  line L645 (97.8199, 0.125) -> (98.5387, 2.1)
  line L646 (99.3816, 2.1) -> (100.1004, 0.125)
  line L647 (98.9602, 2.1) -> (98.9602, 0) construction
  line L648 (98.5387, 2.1) -> (99.3816, 2.1)
  line L649 (97.6414, 0) -> (100.279, 0) construction
  arc A161 (97.6414, 0) -> (97.8199, 0.125) centre (97.6414, 0.19) ccw
  line L650 (97.3894, 0) -> (97.6414, 0)
  line L651 (103.4206, 0) -> (103.6726, 0)
  arc A162 (103.242, 0.125) -> (103.4206, 0) centre (103.4206, 0.19) ccw
  line L652 (101.3164, 1.1) -> (102.8872, 1.1) construction
  line L653 (100.9615, 0.125) -> (101.6803, 2.1)
  line L654 (102.5232, 2.1) -> (103.242, 0.125)
  line L655 (102.1018, 2.1) -> (102.1018, 0) construction
  line L656 (101.6803, 2.1) -> (102.5232, 2.1)
  line L657 (100.783, 0) -> (103.4206, 0) construction
  arc A163 (100.783, 0) -> (100.9615, 0.125) centre (100.783, 0.19) ccw
  line L658 (100.531, 0) -> (100.783, 0)
  line L659 (106.5622, 0) -> (106.8142, 0)
  arc A164 (106.3836, 0.125) -> (106.5622, 0) centre (106.5622, 0.19) ccw
  line L660 (104.458, 1.1) -> (106.0288, 1.1) construction
  line L661 (104.1031, 0.125) -> (104.8219, 2.1)
  line L662 (105.6648, 2.1) -> (106.3836, 0.125)
  line L663 (105.2434, 2.1) -> (105.2434, 0) construction
  line L664 (104.8219, 2.1) -> (105.6648, 2.1)
  line L665 (103.9245, 0) -> (106.5622, 0) construction
  arc A165 (103.9245, 0) -> (104.1031, 0.125) centre (103.9245, 0.19) ccw
  line L666 (103.6726, 0) -> (103.9245, 0)
  line L667 (109.7038, 0) -> (109.9557, 0)
  arc A166 (109.5252, 0.125) -> (109.7038, 0) centre (109.7038, 0.19) ccw
  line L668 (107.5995, 1.1) -> (109.1703, 1.1) construction
  line L669 (107.2447, 0.125) -> (107.9635, 2.1)
  line L670 (108.8064, 2.1) -> (109.5252, 0.125)
  line L671 (108.3849, 2.1) -> (108.3849, 0) construction
  line L672 (107.9635, 2.1) -> (108.8064, 2.1)
  line L673 (107.0661, 0) -> (109.7038, 0) construction
  arc A167 (107.0661, 0) -> (107.2447, 0.125) centre (107.0661, 0.19) ccw
  line L674 (106.8142, 0) -> (107.0661, 0)
  line L675 (112.8453, 0) -> (113.0973, 0)
  arc A168 (112.6668, 0.125) -> (112.8453, 0) centre (112.8453, 0.19) ccw
  line L676 (110.7411, 1.1) -> (112.3119, 1.1) construction
  line L677 (110.3863, 0.125) -> (111.1051, 2.1)
  line L678 (111.948, 2.1) -> (112.6668, 0.125)
  line L679 (111.5265, 2.1) -> (111.5265, 0) construction
  line L680 (111.1051, 2.1) -> (111.948, 2.1)
  line L681 (110.2077, 0) -> (112.8453, 0) construction
  arc A169 (110.2077, 0) -> (110.3863, 0.125) centre (110.2077, 0.19) ccw
  line L682 (109.9557, 0) -> (110.2077, 0)
  line L683 (115.9869, 0) -> (116.2389, 0)
  arc A170 (115.8084, 0.125) -> (115.9869, 0) centre (115.9869, 0.19) ccw
  line L684 (113.8827, 1.1) -> (115.4535, 1.1) construction
  line L685 (113.5279, 0.125) -> (114.2467, 2.1)
  line L686 (115.0896, 2.1) -> (115.8084, 0.125)
  line L687 (114.6681, 2.1) -> (114.6681, 0) construction
  line L688 (114.2467, 2.1) -> (115.0896, 2.1)
  line L689 (113.3493, 0) -> (115.9869, 0) construction
  arc A171 (113.3493, 0) -> (113.5279, 0.125) centre (113.3493, 0.19) ccw
  line L690 (113.0973, 0) -> (113.3493, 0)
  line L691 (153.938, 0) -> (153.938, 3.4)
  line L692 (153.938, 3.4) -> (-153.938, 3.4)
  line L693 (-153.938, 0) -> (-153.938, 3.4)
  line L694 (153.938, 0) -> (-153.938, 0) construction
  line L695 (153.938, 3.4) -> (153.938, -5.9) construction
  line L696 (119.1285, 0) -> (119.3805, 0)
  arc A172 (118.95, 0.125) -> (119.1285, 0) centre (119.1285, 0.19) ccw
  line L697 (117.0243, 1.1) -> (118.5951, 1.1) construction
  line L698 (116.6695, 0.125) -> (117.3883, 2.1)
  line L699 (118.2312, 2.1) -> (118.95, 0.125)
  line L700 (117.8097, 2.1) -> (117.8097, 0) construction
  line L701 (117.3883, 2.1) -> (118.2312, 2.1)
  line L702 (116.4909, 0) -> (119.1285, 0) construction
  arc A173 (116.4909, 0) -> (116.6695, 0.125) centre (116.4909, 0.19) ccw
  line L703 (116.2389, 0) -> (116.4909, 0)
  line L704 (122.2701, 0) -> (122.5221, 0)
  arc A174 (122.0916, 0.125) -> (122.2701, 0) centre (122.2701, 0.19) ccw
  line L705 (120.1659, 1.1) -> (121.7367, 1.1) construction